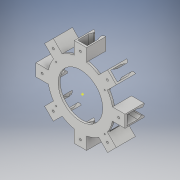
# Autodesk Inventor part: halter
Saved by Autodesk Inventor 2018 (Build 220112000, 112)
## iProperties
Created: 2018-06-16
Part Number: halter
Material: Generisch
Document SubType Name: Modeling
Designer: ich
Density: 1 g/cm^3
Appearance: Vorgabe
Author: ich
Autodesk Inventor part; units mm, degrees
ref_plane "YZ Plane" through (0, 0, 0) normal (1, 0, 0) x (0, 1, 0)
ref_plane "XZ Plane" through (0, 0, 0) normal (0, 1, 0) x (-1, 0, 0)
ref_plane "XY Plane" through (0, 0, 0) normal (0, 0, 1) x (1, 0, 0)
sketch "Skizze1" plane through (0, 0, 0) normal (0, 1, 0) x (-1, 0, 0)
  line L0 (0, 0) -> (100, 0) construction
  line L1 (65.18, 9) -> (46.78, 9)
  line L2 (46.78, 9) -> (46.78, 7)
  line L3 (46.78, 7) -> (65.18, 7)
  line L4 (65.18, 7) -> (65.18, 9)
  dimension "d0" = 100
  dimension "d1" = 18.4
  dimension "d2" = 2
  dimension "d4" = 7
  dimension "d31" = 65.18
  constraints: 10 end point, 2 horizontal, 2 parallel, 1 perpendicular
  measures "d0" distance of L0.start L0.end
  measures "d1" distance of L3.end L2.end
  measures "d2" distance of L3.end L1.start
  measures "d4" distance between parallel lines of L0 L3
  measures "d31" distance from line of L4 L0.start
extrude "Extrusion1" add sketch "Skizze1" along normal blind 25
sketch "Skizze2" plane through (-46.78, 0, 9) normal (1, 0, 0) x (0, 0, -1)
  line L0 (0, 0) -> (2, 0) projected
  line L1 (2, 0) -> (2, 25) projected
  line L2 (0, 25) -> (2, 25) projected
  line L3 (0, 0) -> (0, 25) projected
  line L4 (2, 0) -> (2, 25) projected
  line L5 (2, 21) -> (4, 21)
  line L6 (4, 21) -> (2, 15.505)
  line L7 (2, 22) -> (3.5, 23.5)
  line L8 (3.5, 23.5) -> (2, 25)
  dimension "d9" = 20
  dimension "d10" = 45
  dimension "d12" = 1
  dimension "d13" = 2
  dimension "d14" = 1.5
  dimension "d15" = 45
  constraints: 8 end point, 3 point on line, 1 horizontal
  measures "d9" angle of L1 L6
  measures "d10" angle of L1 L7
  measures "d12" distance of L5.start L7.start
  measures "d13" distance of L5.start L5.end
  measures "d14" distance from line of L1 L7.end
  measures "d15" angle of L1 L8
extrude "Extrusion2" add sketch "Skizze2" against normal up to surface (18.4 mm away) contours L1 L5 L6 | L8 L7 L1
sketch "Skizze3" plane through (-46.78, 21, 7) normal (0, 1, 0) x (1, 0, 0)
  line L0 (-18.4, 2) -> (-18.4, 0) projected
  line L1 (0, 0) -> (-18.4, 0) projected
  line L2 (0, 2) -> (0, 0) projected
  line L3 (0, 2) -> (-18.4, 2) projected
  line L4 (0, 0) -> (-18.4, 0) projected
  line L5 (-18.4, 0) -> (-16.8, 0)
  line L6 (-16.8, 0) -> (-16.8, 2)
  line L7 (-16.8, 2) -> (-18.4, 2)
  line L8 (-18.4, 2) -> (-18.4, 0)
  line L9 (0, 2) -> (0, 0) projected
  line L10 (0, 2) -> (-18.4, 2) projected
  line L11 (0, 0) -> (-1.6, 0)
  line L12 (-1.6, 0) -> (-1.6, 2)
  line L13 (-1.6, 2) -> (0, 2)
  line L14 (0, 2) -> (0, 0)
  point P0 (46.78, 7)
  dimension "d18" = 1.6
  dimension "d19" = 1.6
  dimension "d62" = 15.2
  dimension "d63" = 18.4
  constraints: 16 end point, 4 parallel, 2 horizontal, 2 perpendicular, 2 point on line
  measures "d18" distance between parallel lines of L0 L6
  measures "d19" distance between parallel lines of L2 L12
  measures "d62" distance between parallel lines of L12 L6
  measures "d63" distance between parallel lines of L2 L0
extrude "Extrusion3" add sketch "Skizze3" along normal up to surface contours L3 L6 L1 L0 | L3 L2 L1 L12 surface through (-46.78, 25, 7) normal (0, 0.7071, -0.7071)
mirror "Spiegeln1" about plane through (0, 0, 0) normal (0, 0, 1)
sketch "Skizze4" plane through (-65.18, 0, -9) normal (0, -1, 0) x (1, 0, 0)
  line L0 (0, 0) -> (18.4, 0) projected
  line L1 (18.4, 0) -> (18.4, 2) projected
  line L2 (18.4, 2) -> (0, 2) projected
  line L3 (0, 2) -> (0, 0) projected
  arc A0 (18.4, 0) -> (18.4, 18) centre (65.18, 9) ccw
  line L4 (0, 18) -> (18.4, 18) projected
  line L5 (0, 16) -> (0, 18) projected
  line L6 (18.4, 16) -> (0, 16) projected
  line L7 (18.4, 18) -> (18.4, 16) projected
  line L8 (18.4, 0) -> (0, 0)
  line L9 (0, 18) -> (18.4, 18) projected
  line L10 (0, 0) -> (0, 18)
  line L11 (0, 18) -> (18.4, 18)
  constraints: 6 end point, 3 point on circle, 2 point on line, 1 centre point, 1 coincident, 1 collinear, 1 horizontal, 1 vertical
extrude "Extrusion4" add sketch "Skizze4" along normal blind 3
pattern_circular "Runde Anordnung1" count 8 over 360 about axis through (0, -10, 0) along (0, 1, 0)
sketch "Skizze5" plane through (-65.18, 0, -9) normal (0, 1, 0) x (1, 0, 0)
  line L0 (25.18, -38.25) -> (105.18, -38.25)
  line L1 (105.18, -38.25) -> (105.18, 26.75)
  line L2 (105.18, 26.75) -> (25.18, 26.75)
  line L3 (25.18, 26.75) -> (25.18, -38.25)
  line L4 (65.18, -9) -> (65.18, -5.75) construction
  line L5 (65.18, -5.75) -> (25.18, 26.75) construction
  line L6 (65.18, -5.75) -> (105.18, -38.25) construction
  line L7 (105.18, 26.75) -> (65.18, -5.75) construction
  dimension "d29" = 80
  dimension "d30" = 65
  dimension "d54" = 3.25
  constraints: 16 end point, 2 equal length, 2 parallel, 2 perpendicular, 1 horizontal, 1 vertical
  measures "d29" distance of L1.end L2.end
  measures "d30" distance of L2.end L0.start
  measures "d54" distance of L4.start L4.end
extrude "Extrusion5" cut sketch "Skizze5" along normal through all
sketch "Skizze6" plane through (-65.18, 0, -9) normal (0, 1, 0) x (1, 0, 0)
  line L0 (29.62, -33.69) -> (100.74, -33.69) construction
  line L1 (100.74, -33.69) -> (100.74, 22.19) construction
  line L2 (100.74, 22.19) -> (29.62, 22.19) construction
  line L3 (29.62, 22.19) -> (29.62, -33.69) construction
  circle A0 centre (29.62, -33.69) radius 2.5
  circle A1 centre (29.62, 22.19) radius 2.5
  circle A2 centre (100.74, 22.19) radius 2.5
  circle A3 centre (100.74, -33.69) radius 2.5
  line L4 (65.18, -5.75) -> (65.18, -9) construction
  line L5 (100.74, -33.69) -> (65.18, -5.75) construction
  line L6 (65.18, -5.75) -> (100.74, 22.19) construction
  line L7 (65.18, -5.75) -> (29.62, 22.19) construction
  dimension "d34" = 71.12
  dimension "d35" = 55.88
  dimension "d36" = 5
  dimension "d37" = 5
  dimension "d38" = 5
  dimension "d39" = 5
  dimension "d55" = 3.25
  constraints: 16 end point, 4 centre point, 4 coincident, 2 equal length, 2 parallel, 2 perpendicular, 1 horizontal, 1 vertical
  measures "d34" distance of L1.end L2.end
  measures "d35" distance of L2.end L0.start
  measures "d36" diameter of A0
  measures "d37" diameter of A1
  measures "d38" diameter of A2
  measures "d39" diameter of A3
  measures "d55" distance of L4.start L4.end
extrude "Extrusion6" add sketch "Skizze6" along normal blind 3
sketch "Skizze7" plane through (-35.56, 3, 24.69) normal (0, 1, 0) x (1, 0, 0)
  circle A0 centre (0, 0) radius 2.5 projected
  circle A1 centre (0, 55.88) radius 2.5 projected
  circle A2 centre (71.12, 55.88) radius 2.5 projected
  circle A3 centre (71.12, 0) radius 2.5 projected
  circle A4 centre (0, 0) radius 1.4
  circle A5 centre (0, 55.88) radius 1.4
  circle A6 centre (71.12, 55.88) radius 1.4
  circle A7 centre (71.12, 0) radius 1.4
  point P0 (35.56, 24.69)
  dimension "d42" = 2.8
  dimension "d43" = 2.8
  dimension "d44" = 2.8
  dimension "d45" = 2.8
  constraints: 4 centre point, 4 coincident
  measures "d42" diameter of A4
  measures "d43" diameter of A5
  measures "d44" diameter of A6
  measures "d45" diameter of A7
extrude "Extrusion7" add sketch "Skizze7" along normal blind 1.2 contours A4 | A5 | A6 | A7
sketch "Skizze8" plane through (-35.56, 4.2, 24.69) normal (0, 1, 0) x (1, 0, 0)
  circle A0 centre (0, 0) radius 1.4 projected
  circle A1 centre (0, 55.88) radius 1.4 projected
  circle A2 centre (71.12, 55.88) radius 1.4 projected
  circle A3 centre (71.12, 0) radius 1.4 projected
  circle A4 centre (0, 0) radius 1
  circle A5 centre (0, 55.88) radius 1.4 projected
  circle A6 centre (0, 55.88) radius 1
  circle A7 centre (71.12, 55.88) radius 2.5 projected
  circle A8 centre (71.12, 55.88) radius 1
  circle A9 centre (71.12, 0) radius 1
  point P0 (35.56, 24.69)
  dimension "d48" = 2
  dimension "d49" = 2
  dimension "d50" = 2
  dimension "d51" = 2
  constraints: 4 centre point, 4 coincident
  measures "d48" diameter of A4
  measures "d49" diameter of A6
  measures "d50" diameter of A8
  measures "d51" diameter of A9
extrude "Extrusion8" cut sketch "Skizze8" against normal through all contours A4 | A6 | A8 | A9
chamfer "Fase1" distance 1.977 angle 45 1 edges at (-40, 12.5, 29.25)
chamfer "Fase2" distance 1.977 angle 45 1 edges at (40, 12.5, 29.25)
sketch "Skizze9" plane through (-65.18, 0, -9) normal (0, 1, 0) x (1, 0, 0)
  line L0 (103.7662, -37.6868) -> (105.18, -36.273) projected
  line L1 (105.18, -36.273) -> (105.18, -36.2721) projected
  line L2 (104.6224, -35.7145) -> (105.18, -36.2721) projected
  arc A0 (104.6224, -35.7145) -> (111.96, -18) centre (65.18, -9) ccw projected
  line L3 (111.96, -18) -> (111.96, -16) projected
  line L4 (111.96, -16) -> (130.36, -16) projected
  line L5 (130.36, -2) -> (130.36, -16) projected
  line L6 (130.36, -2) -> (111.96, -2) projected
  line L7 (111.96, -2) -> (111.96, 0) projected
  arc A1 (111.96, 0) -> (104.6224, 17.7145) centre (65.18, -9) ccw projected
  line L8 (105.18, 18.2721) -> (104.6224, 17.7145) projected
  line L9 (105.18, 18.2721) -> (105.18, 21.1005) projected
  line L10 (105.18, 21.1005) -> (116.219, 32.1395) projected
  line L11 (106.3195, 42.039) -> (116.219, 32.1395) projected
  line L12 (106.3195, 42.039) -> (93.3087, 29.0282) projected
  line L13 (93.3087, 29.0282) -> (91.8945, 30.4424) projected
  arc A2 (91.8945, 30.4424) -> (74.18, 37.78) centre (65.18, -9) ccw projected
  line L14 (74.18, 37.78) -> (72.18, 37.78) projected
  line L15 (72.18, 37.78) -> (72.18, 56.18) projected
  line L16 (58.18, 56.18) -> (72.18, 56.18) projected
  line L17 (58.18, 56.18) -> (58.18, 37.78) projected
  line L18 (58.18, 37.78) -> (56.18, 37.78) projected
  arc A3 (56.18, 37.78) -> (38.4655, 30.4424) centre (65.18, -9) ccw projected
  line L19 (38.4655, 30.4424) -> (37.0513, 29.0282) projected
  line L20 (37.0513, 29.0282) -> (24.0405, 42.039) projected
  line L21 (14.141, 32.1395) -> (24.0405, 42.039) projected
  line L22 (14.141, 32.1395) -> (25.18, 21.1005) projected
  line L23 (25.18, 21.1005) -> (25.18, 18.2721) projected
  line L24 (25.7376, 17.7145) -> (25.18, 18.2721) projected
  arc A4 (25.7376, 17.7145) -> (18.4, 0) centre (65.18, -9) ccw projected
  line L25 (18.4, 0) -> (18.4, -2) projected
  line L26 (18.4, -2) -> (0, -2) projected
  line L27 (0, -16) -> (0, -2) projected
  line L28 (18.4, -16) -> (0, -16) projected
  line L29 (18.4, -18) -> (18.4, -16) projected
  arc A5 (18.4, -18) -> (25.7376, -35.7145) centre (65.18, -9) ccw projected
  line L30 (25.18, -36.2721) -> (25.7376, -35.7145) projected
  line L31 (25.18, -36.2721) -> (25.18, -36.273) projected
  line L32 (25.18, -36.273) -> (26.5938, -37.6868) projected
  line L33 (26.5938, -37.6868) -> (14.141, -50.1395) projected
  line L34 (24.0405, -60.039) -> (14.141, -50.1395) projected
  line L35 (24.0405, -60.039) -> (37.0513, -47.0282) projected
  line L36 (37.0513, -47.0282) -> (38.4655, -48.4424) projected
  arc A6 (38.4655, -48.4424) -> (56.18, -55.78) centre (65.18, -9) ccw projected
  line L37 (56.18, -55.78) -> (58.18, -55.78) projected
  line L38 (58.18, -55.78) -> (58.18, -74.18) projected
  line L39 (72.18, -74.18) -> (58.18, -74.18) projected
  line L40 (72.18, -74.18) -> (72.18, -55.78) projected
  line L41 (72.18, -55.78) -> (74.18, -55.78) projected
  arc A7 (74.18, -55.78) -> (91.8945, -48.4424) centre (65.18, -9) ccw projected
  line L42 (91.8945, -48.4424) -> (93.3087, -47.0282) projected
  line L43 (93.3087, -47.0282) -> (106.3195, -60.039) projected
  line L44 (116.219, -50.1395) -> (106.3195, -60.039) projected
  line L45 (116.219, -50.1395) -> (103.7662, -37.6868) projected
  circle A8 centre (100.74, -33.69) radius 2.5 projected
  circle A9 centre (29.62, 22.19) radius 2.5 projected
  circle A10 centre (29.62, -33.69) radius 2.5 projected
  circle A11 centre (100.74, 22.19) radius 2.5 projected
  line L46 (0, -18) -> (18.4, 0) construction
  line L47 (0, -18) -> (18.4, -18) construction
  line L48 (18.4, -18) -> (0, 0) construction
  circle A12 centre (9.2, -9) radius 1.5
  circle A13 centre (65.18, -9) radius 32.6379
  dimension "d64" = 3
  dimension "d65" = 15
  constraints: 4 end point, 2 centre point, 2 midpoint, 1 coincident, 1 point on line
  measures "d64" diameter of A12
  measures "d65" radial gap between concentric circles of A4 A13
extrude "Extrusion9" cut sketch "Skizze9" against normal through all contours A12 | A13
pattern_circular "Runde Anordnung2" count 8 over 360 about axis through (0, -10, 0) along (0, 1, 0) of "Extrusion9"
equation "\"d19\" = d18"
equation "\"d43\" = d42"
equation "\"d44\" = d42"
equation "\"d45\" = d42"
